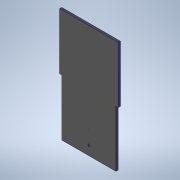
# Autodesk Inventor part: Board
Saved by Autodesk Inventor 2020 (Build 240168000, 168)
## iProperties
Created: 2019-09-17
Part Number: Board
Material: 일반
Document SubType Name: Modeling
Designer: Knowblesse
Density: 1 g/cm^3
Appearance: 기본값
Author: Knowblesse
Autodesk Inventor part; units mm, degrees
ref_plane "YZ Plane" through (0, 0, 0) normal (1, 0, 0) x (0, 1, 0)
ref_plane "XZ Plane" through (0, 0, 0) normal (0, 1, 0) x (-1, 0, 0)
ref_plane "XY Plane" through (0, 0, 0) normal (0, 0, 1) x (1, 0, 0)
sketch "스케치1" plane through (0, 0, 0) normal (0, 0, 1) x (1, 0, 0)
  line L0 (0, 0) -> (240, 0)
  line L1 (240, 0) -> (240, 250)
  line L2 (240, 250) -> (250, 250)
  line L3 (250, 250) -> (250, 500)
  line L4 (250, 500) -> (-10, 500)
  line L5 (-10, 500) -> (-10, 250)
  line L6 (-10, 250) -> (0, 250)
  line L7 (0, 250) -> (0, 0)
  dimension "d0" = 250
  dimension "d1" = 10
  dimension "d2" = 250
  dimension "d3" = 10
  dimension "d4" = 240
  constraints: 16 end point, 6 perpendicular, 2 point on line, 1 horizontal
  measures "d0" distance of L0.end L1.end
  measures "d1" distance of L1.end L2.end
  measures "d2" distance of L2.end L3.end
  measures "d3" distance of L5.end L6.end
  measures "d4" distance between parallel lines of L7 L1
extrude "돌출1" add sketch "스케치1" along normal blind 10
sketch "스케치2" plane through (0, 0, 10) normal (0, 0, 1) x (1, 0, 0)
  line L0 (118, 45) -> (122, 45)
  line L1 (122, 45) -> (122, 35)
  line L2 (122, 35) -> (118, 35)
  line L3 (118, 35) -> (118, 45)
  line L4 (0, 0) -> (240, 0) projected
  point P0 (120, 35)
  point P1 (120, 0)
  dimension "d7" = 35
  dimension "d8" = 10
  dimension "d9" = 4
  constraints: 8 end point, 2 midpoint, 2 parallel, 1 horizontal, 1 perpendicular, 1 vertical alignment
  measures "d7" distance between parallel lines of L2 L4
  measures "d8" distance of L0.end L1.end
  measures "d9" distance between parallel lines of L3 L1
extrude "돌출2" cut sketch "스케치2" against normal blind 10
sketch "스케치3" plane through (0, 0, 10) normal (0, 0, 1) x (1, 0, 0)
  line L0 (118, 45) -> (122, 45) projected
  line L1 (0, 0) -> (240, 0) projected
  point P0 (120, 100)
  point P1 (120, 45)
  dimension "d12" = 100
  constraints: 1 midpoint, 1 vertical alignment
  measures "d12" distance from line of point (120, 100) L1
hole "구멍1" at (120, 100, 10) direction (0, 0, -1) diameter 1 end through all
